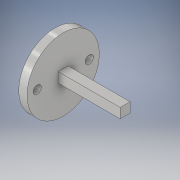
# Autodesk Inventor part: vex servo addapter
Saved by Autodesk Inventor 2019 (Build 230136000, 136)
## iProperties
Created: 2019-02-14
Part Number: vex servo addapter
Material: Aluminum 6061
Document SubType Name: Modeling
Designer: User
Density: 2.7 g/cm^3
Appearance: Aluminum - Polished
Author: User
Autodesk Inventor part; units mm, degrees
ref_plane "YZ Plane" through (0, 0, 0) normal (1, 0, 0) x (0, 1, 0)
ref_plane "XZ Plane" through (0, 0, 0) normal (0, 1, 0) x (-1, 0, 0)
ref_plane "XY Plane" through (0, 0, 0) normal (0, 0, 1) x (1, 0, 0)
sketch "Sketch1" plane through (0, 0, 0) normal (1, 0, 0) x (0, 1, 0)
  circle A0 centre (0, 0) radius 11.1125
  dimension "d0" = 22.225
  constraints: 1 centre point, 1 coincident
  measures "d0" diameter of A0
extrude "Extrusion1" add sketch "Sketch1" along normal blind 2.54
sketch "Sketch2" plane through (2.54, 0, 0) normal (1, 0, 0) x (0, 0, -1)
  line L0 (-1.524, 1.524) -> (1.524, 1.524)
  line L1 (1.524, 1.524) -> (1.524, -1.524)
  line L2 (1.524, -1.524) -> (-1.524, -1.524)
  line L3 (-1.524, -1.524) -> (-1.524, 1.524)
  point P0 (0, 0)
  dimension "d3" = 3.048
  dimension "d4" = 3.048
  dimension "d5" = 1.524
  dimension "d6" = 1.524
  constraints: 8 end point, 2 parallel, 1 horizontal, 1 perpendicular
  measures "d3" distance of L1.end L2.end
  measures "d4" distance of L0.end L1.end
  measures "d5" distance from line of L2 point (0, 0)
  measures "d6" distance from line of L3 point (0, 0)
extrude "Extrusion2" add sketch "Sketch2" along normal blind 19.05
sketch "Sketch3" plane through (0, 0, 0) normal (-1, 0, 0) x (0, 0, 1)
  point P0 (0, 0)
  point P1 (-8.001, 0)
  point P2 (8.001, 0)
  dimension "d9" = 16.002
  dimension "d10" = 8.001
  measures "d9" distance of point (8.001, 0) point (-8.001, 0)
  measures "d10" distance of point (-8.001, 0) point (0, 0)
hole "Hole1" at (0, 0, 8.001) at (0, 0, -8.001) direction (1, 0, 0) diameter 2.4892 depth 2.54
equation "\"d4\" = d3"
equation "\"d5\" = 0.5 * d4"
equation "\"d6\" = 0.5 * d3"
equation "\"d10\" = 0.5 * d9"
body "Solid1"
